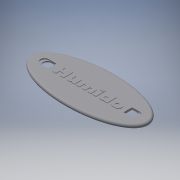
# Autodesk Inventor part: Top Lid
Saved by Autodesk Inventor 2016 (Build 200138000, 138)
## iProperties
Created: 2018-11-09
Part Number: Top Lid
Material: Generic
Document SubType Name: Modeling
Designer: Justin
Density: 1 g/cm^3
Appearance: Default
Author: Justin
Autodesk Inventor part; units mm, degrees
ref_plane "YZ Plane" through (0, 0, 0) normal (1, 0, 0) x (0, 1, 0)
ref_plane "XY Plane" through (0, 0, 0) normal (0, 0, 1) x (1, 0, 0)
ref_plane "XZ .125" through (0, -3.175, 0) normal (0, 1, 0) x (-1, 0, 0)
sketch "Sketch1" plane through (0, 0, 0) normal (0, 1, 0) x (-1, 0, 0)
  ellipse E0 centre (0, 0) end of major axis (-44.7802, 0) minor radius 19.05
  dimension "d0" = 44.7802
  dimension "d1" = 19.05
  constraints: 1 coincident, 2 other
extrude "Extrusion1" add sketch "Sketch1" against normal blind 3.175
fillet "Fillet1" radius 1.5875 2 edges at (-44.7802, -3.175, 0) (-44.7802, 0, 0)
sketch "Sketch5" plane through (0, 0, 0) normal (0, 1, 0) x (-1, 0, 0)
  line L0 (25.1643, 3.6662) -> (25.1643, -3.4417)
  line L1 (25.1643, -3.4417) -> (22.4105, -3.4417)
  line L2 (22.4105, -3.4417) -> (22.4105, -0.9811)
  line L3 (22.4105, -0.9811) -> (19.2675, -0.9811)
  line L4 (19.2675, -0.9811) -> (19.2675, -3.4417)
  line L5 (19.2675, -3.4417) -> (16.5137, -3.4417)
  line L6 (16.5137, -3.4417) -> (16.5137, 3.6662)
  line L7 (16.5137, 3.6662) -> (19.2675, 3.6662)
  line L8 (19.2675, 3.6662) -> (19.2675, 0.7923)
  line L9 (19.2675, 0.7923) -> (22.4105, 0.7923)
  line L10 (22.4105, 0.7923) -> (22.4105, 3.6662)
  line L11 (22.4105, 3.6662) -> (25.1643, 3.6662)
  spline S0 degree 3 poles (10.5976, 3.0943) (10.9244, 3.325) (11.2665, 3.4964) (11.6237, 3.6085) knots 0 0 0 0 1 1 1 1
  line L12 (10.5976, 3.0943) -> (10.9244, 3.325) construction
  line L13 (10.9244, 3.325) -> (11.2665, 3.4964) construction
  line L14 (11.2665, 3.4964) -> (11.6237, 3.6085) construction
  spline S1 degree 3 poles (11.6237, 3.6085) (11.981, 3.7207) (12.3646, 3.7768) (12.7747, 3.7768) (13.5821, 3.7768) (14.1725, 3.5709) (14.5457, 3.1592) knots 1 1 1 1 2 2 2 3 3 3 3
  line L15 (11.6237, 3.6085) -> (11.981, 3.7207) construction
  line L16 (11.981, 3.7207) -> (12.3646, 3.7768) construction
  line L17 (12.3646, 3.7768) -> (12.7747, 3.7768) construction
  line L18 (12.7747, 3.7768) -> (13.5821, 3.7768) construction
  line L19 (13.5821, 3.7768) -> (14.1725, 3.5709) construction
  line L20 (14.1725, 3.5709) -> (14.5457, 3.1592) construction
  spline S2 degree 3 poles (14.5457, 3.1592) (14.919, 2.7476) (15.1056, 2.0964) (15.1056, 1.2056) knots 3 3 3 3 4 4 4 4
  line L21 (14.5457, 3.1592) -> (14.919, 2.7476) construction
  line L22 (14.919, 2.7476) -> (15.1056, 2.0964) construction
  line L23 (15.1056, 2.0964) -> (15.1056, 1.2056) construction
  line L24 (15.1056, 1.2056) -> (15.1056, -1.8462)
  line L25 (15.1056, -1.8462) -> (12.6449, -1.8462)
  line L26 (12.6449, -1.8462) -> (12.6449, 0.7442)
  spline S3 degree 3 poles (12.6449, 0.7442) (12.6449, 1.1544) (12.5793, 1.4371) (12.4479, 1.5925) knots 7 7 7 7 8 8 8 8
  line L27 (12.6449, 0.7442) -> (12.6449, 1.1544) construction
  line L28 (12.6449, 1.1544) -> (12.5793, 1.4371) construction
  line L29 (12.5793, 1.4371) -> (12.4479, 1.5925) construction
  spline S4 degree 3 poles (12.4479, 1.5925) (12.3166, 1.748) (12.0875, 1.8256) (11.7607, 1.8256) (11.3986, 1.8256) (11.1143, 1.739) (10.9076, 1.566) (10.701, 1.393) (10.5976, 1.1544) (10.5976, 0.85) knots 8 8 8 8 9 9 9 10 10 10 11 11 11 11
  line L30 (12.4479, 1.5925) -> (12.3166, 1.748) construction
  line L31 (12.3166, 1.748) -> (12.0875, 1.8256) construction
  line L32 (12.0875, 1.8256) -> (11.7607, 1.8256) construction
  line L33 (11.7607, 1.8256) -> (11.3986, 1.8256) construction
  line L34 (11.3986, 1.8256) -> (11.1143, 1.739) construction
  line L35 (11.1143, 1.739) -> (10.9076, 1.566) construction
  line L36 (10.9076, 1.566) -> (10.701, 1.393) construction
  line L37 (10.701, 1.393) -> (10.5976, 1.1544) construction
  line L38 (10.5976, 1.1544) -> (10.5976, 0.85) construction
  line L39 (10.5976, 0.85) -> (10.5976, -1.8462)
  line L40 (10.5976, -1.8462) -> (8.137, -1.8462)
  line L41 (8.137, -1.8462) -> (8.137, 3.6662)
  line L42 (8.137, 3.6662) -> (10.5976, 3.6662)
  line L43 (10.5976, 3.6662) -> (10.5976, 3.0943)
  line L44 (6.8394, 3.6662) -> (6.8394, -1.8462)
  line L45 (6.8394, -1.8462) -> (4.398, -1.8462)
  line L46 (4.398, -1.8462) -> (4.398, -1.2743)
  spline S5 degree 3 poles (4.398, -1.2743) (4.0712, -1.5081) (3.7365, -1.6795) (3.3936, -1.7885) knots 3 3 3 3 4 4 4 4
  line L47 (4.398, -1.2743) -> (4.0712, -1.5081) construction
  line L48 (4.0712, -1.5081) -> (3.7365, -1.6795) construction
  line L49 (3.7365, -1.6795) -> (3.3936, -1.7885) construction
  spline S6 degree 3 poles (3.3936, -1.7885) (3.0508, -1.8974) (2.6807, -1.9519) (2.2834, -1.9519) (1.8382, -1.9519) (1.4648, -1.8726) (1.1637, -1.714) knots 4 4 4 4 5 5 5 6 6 6 6
  line L50 (3.3936, -1.7885) -> (3.0508, -1.8974) construction
  line L51 (3.0508, -1.8974) -> (2.6807, -1.9519) construction
  line L52 (2.6807, -1.9519) -> (2.2834, -1.9519) construction
  line L53 (2.2834, -1.9519) -> (1.8382, -1.9519) construction
  line L54 (1.8382, -1.9519) -> (1.4648, -1.8726) construction
  line L55 (1.4648, -1.8726) -> (1.1637, -1.714) construction
  spline S7 degree 3 poles (1.1637, -1.714) (0.8626, -1.5554) (0.6046, -1.3047) (0.3899, -0.9619) knots 6 6 6 6 7 7 7 7
  line L56 (1.1637, -1.714) -> (0.8626, -1.5554) construction
  line L57 (0.8626, -1.5554) -> (0.6046, -1.3047) construction
  line L58 (0.6046, -1.3047) -> (0.3899, -0.9619) construction
  spline S8 degree 3 poles (0.3899, -0.9619) (0.0279, -1.3014) (-0.3518, -1.5513) (-0.7491, -1.7116) knots 7 7 7 7 8 8 8 8
  line L59 (0.3899, -0.9619) -> (0.0279, -1.3014) construction
  line L60 (0.0279, -1.3014) -> (-0.3518, -1.5513) construction
  line L61 (-0.3518, -1.5513) -> (-0.7491, -1.7116) construction
  spline S9 degree 3 poles (-0.7491, -1.7116) (-1.1463, -1.8718) (-1.5869, -1.9519) (-2.0707, -1.9519) (-2.8493, -1.9519) (-3.4195, -1.7468) (-3.7816, -1.3367) knots 8 8 8 8 9 9 9 10 10 10 10
  line L62 (-0.7491, -1.7116) -> (-1.1463, -1.8718) construction
  line L63 (-1.1463, -1.8718) -> (-1.5869, -1.9519) construction
  line L64 (-1.5869, -1.9519) -> (-2.0707, -1.9519) construction
  line L65 (-2.0707, -1.9519) -> (-2.8493, -1.9519) construction
  line L66 (-2.8493, -1.9519) -> (-3.4195, -1.7468) construction
  line L67 (-3.4195, -1.7468) -> (-3.7816, -1.3367) construction
  spline S10 degree 3 poles (-3.7816, -1.3367) (-4.1437, -0.9266) (-4.3247, -0.2762) (-4.3247, 0.6145) knots 10 10 10 10 11 11 11 11
  line L68 (-3.7816, -1.3367) -> (-4.1437, -0.9266) construction
  line L69 (-4.1437, -0.9266) -> (-4.3247, -0.2762) construction
  line L70 (-4.3247, -0.2762) -> (-4.3247, 0.6145) construction
  line L71 (-4.3247, 0.6145) -> (-4.3247, 3.6662)
  line L72 (-4.3247, 3.6662) -> (-1.8929, 3.6662)
  line L73 (-1.8929, 3.6662) -> (-1.8929, 1.0758)
  spline S11 degree 3 poles (-1.8929, 1.0758) (-1.8929, 0.6721) (-1.8288, 0.391) (-1.7007, 0.2324) knots 14 14 14 14 15 15 15 15
  line L74 (-1.8929, 1.0758) -> (-1.8929, 0.6721) construction
  line L75 (-1.8929, 0.6721) -> (-1.8288, 0.391) construction
  line L76 (-1.8288, 0.391) -> (-1.7007, 0.2324) construction
  spline S12 degree 3 poles (-1.7007, 0.2324) (-1.5725, 0.0738) (-1.3546, -0.0055) (-1.0471, -0.0055) (-0.701, -0.0055) (-0.4302, 0.081) (-0.2349, 0.254) knots 15 15 15 15 16 16 16 17 17 17 17
  line L77 (-1.7007, 0.2324) -> (-1.5725, 0.0738) construction
  line L78 (-1.5725, 0.0738) -> (-1.3546, -0.0055) construction
  line L79 (-1.3546, -0.0055) -> (-1.0471, -0.0055) construction
  line L80 (-1.0471, -0.0055) -> (-0.701, -0.0055) construction
  line L81 (-0.701, -0.0055) -> (-0.4302, 0.081) construction
  line L82 (-0.4302, 0.081) -> (-0.2349, 0.254) construction
  spline S13 degree 3 poles (-0.2349, 0.254) (-0.0394, 0.427) (0.0583, 0.6658) (0.0583, 0.9701) knots 17 17 17 17 18 18 18 18
  line L83 (-0.2349, 0.254) -> (-0.0394, 0.427) construction
  line L84 (-0.0394, 0.427) -> (0.0583, 0.6658) construction
  line L85 (0.0583, 0.6658) -> (0.0583, 0.9701) construction
  line L86 (0.0583, 0.9701) -> (0.0583, 3.6662)
  line L87 (0.0583, 3.6662) -> (2.4468, 3.6662)
  line L88 (2.4468, 3.6662) -> (2.4468, 1.0758)
  spline S14 degree 3 poles (2.4468, 1.0758) (2.4468, 0.6721) (2.511, 0.391) (2.6391, 0.2324) knots 21 21 21 21 22 22 22 22
  line L89 (2.4468, 1.0758) -> (2.4468, 0.6721) construction
  line L90 (2.4468, 0.6721) -> (2.511, 0.391) construction
  line L91 (2.511, 0.391) -> (2.6391, 0.2324) construction
  spline S15 degree 3 poles (2.6391, 0.2324) (2.7672, 0.0738) (2.9868, -0.0055) (3.2975, -0.0055) (3.6404, -0.0055) (3.9095, 0.081) (4.1049, 0.254) knots 22 22 22 22 23 23 23 24 24 24 24
  line L92 (2.6391, 0.2324) -> (2.7672, 0.0738) construction
  line L93 (2.7672, 0.0738) -> (2.9868, -0.0055) construction
  line L94 (2.9868, -0.0055) -> (3.2975, -0.0055) construction
  line L95 (3.2975, -0.0055) -> (3.6404, -0.0055) construction
  line L96 (3.6404, -0.0055) -> (3.9095, 0.081) construction
  line L97 (3.9095, 0.081) -> (4.1049, 0.254) construction
  spline S16 degree 3 poles (4.1049, 0.254) (4.3003, 0.427) (4.398, 0.6658) (4.398, 0.9701) knots 24 24 24 24 25 25 25 25
  line L98 (4.1049, 0.254) -> (4.3003, 0.427) construction
  line L99 (4.3003, 0.427) -> (4.398, 0.6658) construction
  line L100 (4.398, 0.6658) -> (4.398, 0.9701) construction
  line L101 (4.398, 0.9701) -> (4.398, 3.6662)
  line L102 (4.398, 3.6662) -> (6.8394, 3.6662)
  line L103 (-5.6944, -2.2979) -> (-5.6944, -3.6964)
  line L104 (-5.6944, -3.6964) -> (-8.2031, -3.6964)
  line L105 (-8.2031, -3.6964) -> (-8.2031, -2.2979)
  line L106 (-8.2031, -2.2979) -> (-5.6944, -2.2979)
  line L107 (-5.6944, 3.6662) -> (-5.6944, -1.8462)
  line L108 (-5.6944, -1.8462) -> (-8.2031, -1.8462)
  line L109 (-8.2031, -1.8462) -> (-8.2031, 3.6662)
  line L110 (-8.2031, 3.6662) -> (-5.6944, 3.6662)
  line L111 (-16.8008, -3.4994) -> (-16.8008, 3.6662)
  line L112 (-16.8008, 3.6662) -> (-14.4603, 3.6662)
  line L113 (-14.4603, 3.6662) -> (-14.4411, 3.1231)
  spline S17 degree 3 poles (-14.4411, 3.1231) (-14.1432, 3.3507) (-13.8132, 3.5213) (-13.4511, 3.6349) knots 3 3 3 3 4 4 4 4
  line L114 (-14.4411, 3.1231) -> (-14.1432, 3.3507) construction
  line L115 (-14.1432, 3.3507) -> (-13.8132, 3.5213) construction
  line L116 (-13.8132, 3.5213) -> (-13.4511, 3.6349) construction
  spline S18 degree 3 poles (-13.4511, 3.6349) (-13.089, 3.7486) (-12.6901, 3.8056) (-12.2544, 3.8056) (-11.3348, 3.8056) (-10.6012, 3.5421) (-10.0533, 3.015) knots 4 4 4 4 5 5 5 6 6 6 6
  line L117 (-13.4511, 3.6349) -> (-13.089, 3.7486) construction
  line L118 (-13.089, 3.7486) -> (-12.6901, 3.8056) construction
  line L119 (-12.6901, 3.8056) -> (-12.2544, 3.8056) construction
  line L120 (-12.2544, 3.8056) -> (-11.3348, 3.8056) construction
  line L121 (-11.3348, 3.8056) -> (-10.6012, 3.5421) construction
  line L122 (-10.6012, 3.5421) -> (-10.0533, 3.015) construction
  spline S19 degree 3 poles (-10.0533, 3.015) (-9.5055, 2.4881) (-9.2315, 1.7871) (-9.2315, 0.9124) (-9.2315, 0.025) (-9.5079, -0.6799) (-10.0605, -1.2022) knots 6 6 6 6 7 7 7 8 8 8 8
  line L123 (-10.0533, 3.015) -> (-9.5055, 2.4881) construction
  line L124 (-9.5055, 2.4881) -> (-9.2315, 1.7871) construction
  line L125 (-9.2315, 1.7871) -> (-9.2315, 0.9124) construction
  line L126 (-9.2315, 0.9124) -> (-9.2315, 0.025) construction
  line L127 (-9.2315, 0.025) -> (-9.5079, -0.6799) construction
  line L128 (-9.5079, -0.6799) -> (-10.0605, -1.2022) construction
  spline S20 degree 3 poles (-10.0605, -1.2022) (-10.6133, -1.7243) (-11.3573, -1.9855) (-12.2929, -1.9855) (-12.6901, -1.9855) (-13.0562, -1.9366) (-13.3911, -1.839) knots 8 8 8 8 9 9 9 10 10 10 10
  line L129 (-10.0605, -1.2022) -> (-10.6133, -1.7243) construction
  line L130 (-10.6133, -1.7243) -> (-11.3573, -1.9855) construction
  line L131 (-11.3573, -1.9855) -> (-12.2929, -1.9855) construction
  line L132 (-12.2929, -1.9855) -> (-12.6901, -1.9855) construction
  line L133 (-12.6901, -1.9855) -> (-13.0562, -1.9366) construction
  line L134 (-13.0562, -1.9366) -> (-13.3911, -1.839) construction
  spline S21 degree 3 poles (-13.3911, -1.839) (-13.7258, -1.7412) (-14.0422, -1.593) (-14.3402, -1.3944) knots 10 10 10 10 11 11 11 11
  line L135 (-13.3911, -1.839) -> (-13.7258, -1.7412) construction
  line L136 (-13.7258, -1.7412) -> (-14.0422, -1.593) construction
  line L137 (-14.0422, -1.593) -> (-14.3402, -1.3944) construction
  line L138 (-14.3402, -1.3944) -> (-14.3402, -3.4994)
  line L139 (-14.3402, -3.4994) -> (-16.8008, -3.4994)
  spline S22 degree 3 poles (-14.3402, 0.9124) (-14.3402, 0.5408) (-14.2256, 0.2444) (-13.9966, 0.0233) (-13.7675, -0.1977) (-13.4623, -0.3083) (-13.0811, -0.3083) (-12.6997, -0.3083) (-12.3946, -0.1977) (-12.1655, 0.0233) (-11.9364, 0.2444) (-11.8219, 0.5408) (-11.8219, 0.9124) (-11.8219, 1.2809) (-11.9364, 1.5765) (-12.1655, 1.7991) (-12.3946, 2.0218) (-12.6997, 2.1331) (-13.0811, 2.1331) (-13.4623, 2.1331) (-13.7675, 2.0218) (-13.9966, 1.7991) (-14.2256, 1.5765) (-14.3402, 1.2809) (-14.3402, 0.9124) knots 0 0 0 0 1 1 1 2 2 2 3 3 3 4 4 4 5 5 5 6 6 6 7 7 7 8 8 8 8
  line L140 (-14.3402, 0.9124) -> (-14.3402, 0.5408) construction
  line L141 (-14.3402, 0.5408) -> (-14.2256, 0.2444) construction
  line L142 (-14.2256, 0.2444) -> (-13.9966, 0.0233) construction
  line L143 (-13.9966, 0.0233) -> (-13.7675, -0.1977) construction
  line L144 (-13.7675, -0.1977) -> (-13.4623, -0.3083) construction
  line L145 (-13.4623, -0.3083) -> (-13.0811, -0.3083) construction
  line L146 (-13.0811, -0.3083) -> (-12.6997, -0.3083) construction
  line L147 (-12.6997, -0.3083) -> (-12.3946, -0.1977) construction
  line L148 (-12.3946, -0.1977) -> (-12.1655, 0.0233) construction
  line L149 (-12.1655, 0.0233) -> (-11.9364, 0.2444) construction
  line L150 (-11.9364, 0.2444) -> (-11.8219, 0.5408) construction
  line L151 (-11.8219, 0.5408) -> (-11.8219, 0.9124) construction
  line L152 (-11.8219, 0.9124) -> (-11.8219, 1.2809) construction
  line L153 (-11.8219, 1.2809) -> (-11.9364, 1.5765) construction
  line L154 (-11.9364, 1.5765) -> (-12.1655, 1.7991) construction
  line L155 (-12.1655, 1.7991) -> (-12.3946, 2.0218) construction
  line L156 (-12.3946, 2.0218) -> (-12.6997, 2.1331) construction
  line L157 (-12.6997, 2.1331) -> (-13.0811, 2.1331) construction
  line L158 (-13.0811, 2.1331) -> (-13.4623, 2.1331) construction
  line L159 (-13.4623, 2.1331) -> (-13.7675, 2.0218) construction
  line L160 (-13.7675, 2.0218) -> (-13.9966, 1.7991) construction
  line L161 (-13.9966, 1.7991) -> (-14.2256, 1.5765) construction
  line L162 (-14.2256, 1.5765) -> (-14.3402, 1.2809) construction
  line L163 (-14.3402, 1.2809) -> (-14.3402, 0.9124) construction
  spline S23 degree 3 poles (-17.7668, 0.9124) (-17.7668, -0.0231) (-18.1048, -0.748) (-18.7809, -1.2622) (-19.4568, -1.7765) (-20.4117, -2.0336) (-21.6452, -2.0336) (-22.8819, -2.0336) (-23.8358, -1.7772) (-24.5071, -1.2646) (-25.1783, -0.752) (-25.5139, -0.0263) (-25.5139, 0.9124) (-25.5139, 1.848) (-25.1783, 2.5721) (-24.5071, 3.0847) (-23.8358, 3.5974) (-22.8819, 3.8536) (-21.6452, 3.8536) (-20.4117, 3.8536) (-19.4568, 3.5974) (-18.7809, 3.0847) (-18.1048, 2.5721) (-17.7668, 1.848) (-17.7668, 0.9124) knots 0 0 0 0 1 1 1 2 2 2 3 3 3 4 4 4 5 5 5 6 6 6 7 7 7 8 8 8 8
  line L164 (-17.7668, 0.9124) -> (-17.7668, -0.0231) construction
  line L165 (-17.7668, -0.0231) -> (-18.1048, -0.748) construction
  line L166 (-18.1048, -0.748) -> (-18.7809, -1.2622) construction
  line L167 (-18.7809, -1.2622) -> (-19.4568, -1.7765) construction
  line L168 (-19.4568, -1.7765) -> (-20.4117, -2.0336) construction
  line L169 (-20.4117, -2.0336) -> (-21.6452, -2.0336) construction
  line L170 (-21.6452, -2.0336) -> (-22.8819, -2.0336) construction
  line L171 (-22.8819, -2.0336) -> (-23.8358, -1.7772) construction
  line L172 (-23.8358, -1.7772) -> (-24.5071, -1.2646) construction
  line L173 (-24.5071, -1.2646) -> (-25.1783, -0.752) construction
  line L174 (-25.1783, -0.752) -> (-25.5139, -0.0263) construction
  line L175 (-25.5139, -0.0263) -> (-25.5139, 0.9124) construction
  line L176 (-25.5139, 0.9124) -> (-25.5139, 1.848) construction
  line L177 (-25.5139, 1.848) -> (-25.1783, 2.5721) construction
  line L178 (-25.1783, 2.5721) -> (-24.5071, 3.0847) construction
  line L179 (-24.5071, 3.0847) -> (-23.8358, 3.5974) construction
  line L180 (-23.8358, 3.5974) -> (-22.8819, 3.8536) construction
  line L181 (-22.8819, 3.8536) -> (-21.6452, 3.8536) construction
  line L182 (-21.6452, 3.8536) -> (-20.4117, 3.8536) construction
  line L183 (-20.4117, 3.8536) -> (-19.4568, 3.5974) construction
  line L184 (-19.4568, 3.5974) -> (-18.7809, 3.0847) construction
  line L185 (-18.7809, 3.0847) -> (-18.1048, 2.5721) construction
  line L186 (-18.1048, 2.5721) -> (-17.7668, 1.848) construction
  line L187 (-17.7668, 1.848) -> (-17.7668, 0.9124) construction
  spline S24 degree 3 poles (-20.3668, 0.9124) (-20.3668, 1.2905) (-20.4813, 1.5917) (-20.7104, 1.8159) (-20.9395, 2.0403) (-21.2479, 2.1524) (-21.6356, 2.1524) (-22.0232, 2.1524) (-22.3316, 2.0403) (-22.5607, 1.8159) (-22.7898, 1.5917) (-22.9043, 1.2905) (-22.9043, 0.9124) (-22.9043, 0.5312) (-22.7898, 0.2293) (-22.5607, 0.0065) (-22.3316, -0.2161) (-22.0232, -0.3275) (-21.6356, -0.3275) (-21.2479, -0.3275) (-20.9395, -0.2161) (-20.7104, 0.0065) (-20.4813, 0.2293) (-20.3668, 0.5312) (-20.3668, 0.9124) knots 0 0 0 0 1 1 1 2 2 2 3 3 3 4 4 4 5 5 5 6 6 6 7 7 7 8 8 8 8
  line L188 (-20.3668, 0.9124) -> (-20.3668, 1.2905) construction
  line L189 (-20.3668, 1.2905) -> (-20.4813, 1.5917) construction
  line L190 (-20.4813, 1.5917) -> (-20.7104, 1.8159) construction
  line L191 (-20.7104, 1.8159) -> (-20.9395, 2.0403) construction
  line L192 (-20.9395, 2.0403) -> (-21.2479, 2.1524) construction
  line L193 (-21.2479, 2.1524) -> (-21.6356, 2.1524) construction
  line L194 (-21.6356, 2.1524) -> (-22.0232, 2.1524) construction
  line L195 (-22.0232, 2.1524) -> (-22.3316, 2.0403) construction
  line L196 (-22.3316, 2.0403) -> (-22.5607, 1.8159) construction
  line L197 (-22.5607, 1.8159) -> (-22.7898, 1.5917) construction
  line L198 (-22.7898, 1.5917) -> (-22.9043, 1.2905) construction
  line L199 (-22.9043, 1.2905) -> (-22.9043, 0.9124) construction
  line L200 (-22.9043, 0.9124) -> (-22.9043, 0.5312) construction
  line L201 (-22.9043, 0.5312) -> (-22.7898, 0.2293) construction
  line L202 (-22.7898, 0.2293) -> (-22.5607, 0.0065) construction
  line L203 (-22.5607, 0.0065) -> (-22.3316, -0.2161) construction
  line L204 (-22.3316, -0.2161) -> (-22.0232, -0.3275) construction
  line L205 (-22.0232, -0.3275) -> (-21.6356, -0.3275) construction
  line L206 (-21.6356, -0.3275) -> (-21.2479, -0.3275) construction
  line L207 (-21.2479, -0.3275) -> (-20.9395, -0.2161) construction
  line L208 (-20.9395, -0.2161) -> (-20.7104, 0.0065) construction
  line L209 (-20.7104, 0.0065) -> (-20.4813, 0.2293) construction
  line L210 (-20.4813, 0.2293) -> (-20.3668, 0.5312) construction
  line L211 (-20.3668, 0.5312) -> (-20.3668, 0.9124) construction
  point P0 (0, 0)
  constraints: 88 end point, 72 other
extrude "Extrusion2" add sketch "Sketch5" along normal blind 0.381
sketch "Sketch6" plane through (0, -3.175, 0) normal (0, -1, 0) x (1, 0, 0)
  spline S0 degree 5 poles (44.7802, 0) (44.7802, -2.9491) (43.4393, -5.9235) (40.7079, -8.7647) (36.7252, -11.3054) (26.7821, -15.5592) (20.8212, -17.2723) (14.1303, -18.456) (7.0796, -19.0478) (-7.0152, -19.0522) (-14.0593, -18.4646) (-20.7359, -17.2881) (-26.6885, -15.587) (-36.6383, -11.3545) (-40.6357, -8.8231) (-43.3994, -5.9848) (-44.7802, -2.9924) (-44.7802, 2.9924) (-43.3994, 5.9848) (-40.6357, 8.8231) (-36.6383, 11.3545) (-26.6885, 15.587) (-20.7359, 17.2881) (-14.0593, 18.4646) (-7.0152, 19.0522) (7.0796, 19.0478) (14.1303, 18.456) (20.8212, 17.2723) (26.7821, 15.5592) (36.7252, 11.3054) (40.7079, 8.7647) (43.4393, 5.9235) (44.7802, 2.9491) (44.7802, 0) knots 0 0 0 0 0 0 0.125 0.125 0.125 0.125 0.25 0.25 0.25 0.25 0.375 0.375 0.375 0.375 0.5 0.5 0.5 0.5 0.625 0.625 0.625 0.625 0.75 0.75 0.75 0.75 0.875 0.875 0.875 0.875 1 1 1 1 1 1 construction
  spline S1 degree 5 poles (40.9702, 0) (40.9713, -0.6823) (40.8308, -1.3669) (40.5695, -2.0065) (39.6758, -3.625) (38.3928, -4.9746) (37.5219, -5.7393) (35.2475, -7.4546) (32.7493, -8.8287) (31.2258, -9.5552) (27.7251, -11.0195) (24.102, -12.1534) (22.066, -12.6998) (17.6985, -13.7028) (13.271, -14.3974) (10.9149, -14.6878) (6.0985, -15.1298) (1.2638, -15.2768) (-1.1998, -15.2776) (-6.0317, -15.1337) (-10.8457, -14.6953) (-13.1992, -14.4071) (-17.6218, -13.7171) (-21.985, -12.72) (-24.0191, -12.177) (-27.6437, -11.0483) (-31.1471, -9.591) (-32.6746, -8.8665) (-35.1849, -7.494) (-37.4734, -5.7799) (-38.3525, -5.0139) (-39.6523, -3.6572) (-40.5599, -2.0297) (-40.8284, -1.3821) (-41.1125, 0) (-40.8284, 1.3821) (-40.5599, 2.0297) (-39.6523, 3.6572) (-38.3525, 5.0139) (-37.4734, 5.7799) (-35.1849, 7.494) (-32.6746, 8.8665) (-31.1471, 9.591) (-27.6437, 11.0483) (-24.0191, 12.177) (-21.985, 12.72) (-17.6218, 13.7171) (-13.1992, 14.4071) (-10.8457, 14.6953) (-6.0317, 15.1337) (-1.1998, 15.2776) (1.2638, 15.2768) (6.0985, 15.1298) (10.9149, 14.6878) (13.271, 14.3974) (17.6985, 13.7028) (22.066, 12.6998) (24.102, 12.1534) (27.7251, 11.0195) (31.2258, 9.5552) (32.7493, 8.8287) (35.2475, 7.4546) (37.5219, 5.7393) (38.3928, 4.9746) (39.6758, 3.625) (40.5695, 2.0065) (40.8308, 1.3669) (40.9713, 0.6823) (40.9702, 0) knots 0 0 0 0 0 0 0.018466 0.018466 0.018466 0.049772 0.049772 0.049772 0.09536 0.09536 0.09536 0.152341 0.152341 0.152341 0.216522 0.216522 0.216522 0.283132 0.283132 0.283132 0.347236 0.347236 0.347236 0.404145 0.404145 0.404145 0.449803 0.449803 0.449803 0.481315 0.481315 0.481315 0.5 0.5 0.5 0.518685 0.518685 0.518685 0.550197 0.550197 0.550197 0.595855 0.595855 0.595855 0.652764 0.652764 0.652764 0.716868 0.716868 0.716868 0.783478 0.783478 0.783478 0.847659 0.847659 0.847659 0.90464 0.90464 0.90464 0.950228 0.950228 0.950228 0.981534 0.981534 0.981534 1 1 1 1 1 1
  dimension "d10" = 3.81
  constraints: 3 other
extrude "Extrusion3" cut sketch "Sketch6" against normal blind 1.5875
sketch "Sketch7" plane through (0, -1.5875, 0) normal (0, -1, 0) x (1, 0, 0)
  line L0 (0, 26.7828) -> (0, -26.7774) construction
  line L1 (-62.7817, 0) -> (62.7181, 0) construction
  line L2 (28.956, -3.2512) -> (28.956, 3.2512)
  line L3 (28.956, -3.2512) -> (32.6136, -3.2512)
  line L4 (28.956, 3.2512) -> (32.6136, 3.2512)
  arc A0 (32.6136, -3.2512) -> (32.6136, 3.2512) centre (32.6136, 0) ccw
  line L5 (-28.956, -3.2512) -> (-28.956, 3.2512)
  line L6 (-28.956, -3.2512) -> (-32.6136, -3.2512)
  line L7 (-28.956, 3.2512) -> (-32.6136, 3.2512)
  arc A1 (-32.6136, 3.2512) -> (-32.6136, -3.2512) centre (-32.6136, 0) ccw
  point P0 (0, 0)
  point P1 (35.8648, 0)
  point P2 (-35.8648, 0)
  dimension "d14" = 6.5024
  dimension "d15" = 28.956
  dimension "d16" = 6.9088
  constraints: 12 end point, 7 symmetric about line, 5 point on circle, 2 centre point, 2 horizontal, 1 point on line, 1 tangent, 1 vertical, 1 other
  measures "d14" distance of L2.start L2.end
  measures "d15" distance between parallel lines of L0 L2
  measures "d16" distance from line of L2 point (35.865, 0)
extrude "Extrusion4" cut sketch "Sketch7" against normal through all
sketch "Sketch10" plane through (0, 0, 0) normal (0, 1, 0) x (-1, 0, 0)
  line L0 (28.956, -3.2512) -> (28.956, 3.2512) projected
  line L1 (28.956, -3.2512) -> (34.7472, -3.2512)
  line L2 (32.6136, -3.2512) -> (28.956, -3.2512) projected
  line L3 (28.956, 3.2512) -> (34.7472, 3.2512)
  line L4 (28.956, 3.2512) -> (32.6136, 3.2512) projected
  line L5 (28.956, -3.2512) -> (28.956, 3.2512)
  arc A0 (34.7472, -3.2512) -> (34.7472, 3.2512) centre (34.7472, 0) ccw
  line L6 (0, -29.029) -> (0, 41.7031)
  line L7 (-28.956, -3.2512) -> (-28.956, 3.2512)
  line L8 (-28.956, -3.2512) -> (-34.7472, -3.2512)
  line L9 (-32.6136, -3.2512) -> (-28.956, -3.2512)
  line L10 (-28.956, 3.2512) -> (-34.7472, 3.2512)
  line L11 (-28.956, 3.2512) -> (-32.6136, 3.2512)
  line L12 (-28.956, -3.2512) -> (-28.956, 3.2512)
  arc A1 (-34.7472, 3.2512) -> (-34.7472, -3.2512) centre (-34.7472, 0) ccw
  line L13 (-28.956, 3.2512) -> (-28.956, -3.2512) construction
  point P0 (0, 0)
  point P1 (37.9984, 0)
  point P2 (-37.9984, 0)
  dimension "d21" = 9.0424
  constraints: 20 end point, 8 symmetric about line, 5 point on circle, 4 point on line, 2 centre point, 2 collinear, 2 tangent, 1 vertical, 1 other
  measures "d21" distance from line of L0 point (37.998, 0)
extrude "Extrusion5" cut sketch "Sketch10" against normal blind 0.7937
body "Solid1"
